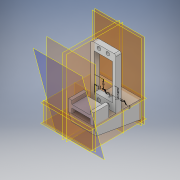
# Autodesk Inventor part: Motor
Saved by Autodesk Inventor 2019.4 (Build 234330000, 330)
## iProperties
Created: 2019-08-20
Part Number: Motor
Material: Genérico
Document SubType Name: Modeling
Designer: Irene
Density: 1 g/cm^3
Appearance: Valor por defecto
Author: Irene
Autodesk Inventor part; units mm, degrees
ref_plane "Plano de trabajo1" through (0, 0, 23) normal (0, 0, 1) x (1, 0, 0)
sketch "Boceto2" plane through (0, 0, 23) normal (0, 0, 1) x (1, 0, 0)
  line L0 (-3, 10) -> (25, 10)
  line L1 (25, 10) -> (25, 65)
  line L2 (23, 67) -> (-1, 67)
  line L3 (-3, 65) -> (-3, 10)
  line L4 (-3, 10) -> (25, 67) construction
  line L5 (25, 10) -> (-3, 67) construction
  line L6 (21.25, 18.406) -> (0.75, 18.406)
  line L7 (0.75, 18.406) -> (0.75, 58.594)
  line L8 (0.75, 58.594) -> (21.25, 58.594)
  line L9 (21.25, 58.594) -> (21.25, 18.406)
  line L10 (21.25, 18.406) -> (0.75, 58.594) construction
  line L11 (0.75, 18.406) -> (21.25, 58.594) construction
  circle A0 centre (6, 63.5) radius 2
  circle A1 centre (16, 63.5) radius 2
  circle A2 centre (6, 13.5) radius 2
  circle A3 centre (16, 13.5) radius 2
  line L12 (25, -6.6) -> (-3, -6.6)
  line L13 (-3, -6.6) -> (-3, 10)
  line L14 (-3, 10) -> (25, 10)
  line L15 (25, 10) -> (25, -6.6)
  line L16 (25, -6.6) -> (-3, 10) construction
  line L17 (-3, -6.6) -> (25, 10) construction
  arc A4 (-1, 67) -> (-3, 65) centre (-1, 65) ccw
  arc A5 (25, 65) -> (23, 67) centre (23, 65) ccw
  point P0 (0, 0)
  point P1 (11, 38.5)
  point P2 (11, 1.7)
  dimension "d5" = 28
  dimension "d6" = 57
  dimension "d9" = 67
  dimension "d10" = 10
  dimension "d12" = 25
  dimension "d13" = 20.5
  dimension "d14" = 40.188
  dimension "d15" = 4
  dimension "d16" = 4
  dimension "d17" = 4
  dimension "d18" = 4
  dimension "d21" = 10
  dimension "d22" = 10
  dimension "d23" = 7
  dimension "d26" = 3.5
  dimension "d27" = 3.5
  dimension "d28" = 3.5
  dimension "d29" = 3.5
  dimension "d38" = 28
  dimension "d39" = 16.6
  dimension "d40" = 25
  dimension "d41" = 10
  dimension "d82" = 2
  dimension "d84" = 7
  dimension "d85" = 9
  constraints: 36 end point, 6 centre point, 6 midpoint, 6 parallel, 4 point on circle, 4 point on line, 4 tangent, 3 horizontal, 3 perpendicular, 1 equal radius
  measures "d5" distance of L5.end L4.end
  measures "d6" distance of L4.end L0.end
  measures "d9" distance from line of point (0, 0) L2
  measures "d10" distance from line of L0 point (0, 0)
  measures "d12" distance from line of L1 point (0, 0)
  measures "d13" distance of L7.end L8.end
  measures "d14" distance of L8.end L6.start
  measures "d15" diameter of A0
  measures "d16" diameter of A1
  measures "d17" diameter of A2
  measures "d18" diameter of A3
  measures "d21" distance of A1.centre A0.centre
  measures "d22" distance of A2.centre A3.centre
  measures "d23" distance edge to line of A2 L3
  measures "d26" distance from line of A2.centre L0
  measures "d27" distance from line of A3.centre L0
  measures "d28" distance from line of A1.centre L2
  measures "d29" distance from line of L2 A0.centre
  measures "d38" distance of L13.end L14.end
  measures "d39" distance of L12.end L13.end
  measures "d40" distance from line of L15 point (0, 0)
  measures "d41" distance from line of L14 point (0, 0)
  measures "d82" radius of A4
  measures "d84" distance edge to line of A1 L1
  measures "d85" distance from line of A0.centre L3
ref_plane "Plano de trabajo2" through (0, 0, 58) normal (0, 0, 1) x (1, 0, 0)
sketch "Boceto3" plane through (0, 0, 58) normal (0, 0, 1) x (1, 0, 0)
  line L0 (25, 0) -> (-3, 0)
  line L1 (-3, 0) -> (-3, 10)
  line L2 (-3, 10) -> (25, 10)
  line L3 (25, 10) -> (25, 0)
  line L4 (25, 0) -> (-3, 10) construction
  line L5 (-3, 0) -> (25, 10) construction
  point P0 (0, 0)
  point P1 (11, 5)
  dimension "d31" = 28
  dimension "d32" = 10
  dimension "d35" = 10
  dimension "d36" = 25
  constraints: 12 end point, 2 midpoint, 2 parallel, 1 horizontal, 1 perpendicular
  measures "d31" distance of L1.end L2.end
  measures "d32" distance of L0.end L1.end
  measures "d35" distance from line of L2 point (0, 0)
  measures "d36" distance from line of L3 point (0, 0)
ref_plane "Plano de trabajo3" through (25, 10, 0) normal (0, 0, 1) x (-1, 0, 0)
sketch "Boceto4" plane through (25, 10, 0) normal (0, 0, 1) x (-1, 0, 0)
  line L0 (0, 0) -> (50, 0)
  line L1 (50, 0) -> (50, 20)
  line L2 (50, 20) -> (0, 20)
  line L3 (0, 20) -> (0, 0)
  line L4 (0, 0) -> (50, 20) construction
  line L5 (50, 0) -> (0, 20) construction
  line L6 (0, 20) -> (0, 0)
  line L7 (28, 0) -> (28, 20)
  point P0 (0, 0)
  dimension "d42" = 50
  dimension "d43" = 20
  dimension "d44" = 50
  dimension "d46" = 28
  constraints: 16 end point, 2 horizontal, 2 parallel, 2 perpendicular, 2 point on line, 2 vertical, 2 other
  measures "d42" distance of L2.end L1.end
  measures "d43" distance of L2.end L0.start
  measures "d44" distance between parallel lines of L1 L6
  measures "d46" distance between parallel lines of L7 L3
ref_plane "Plano de trabajo4" through (25, 10, 0) normal (0, 0, 1) x (-1, 0, 0)
sketch "Boceto5" plane through (25, 10, 0) normal (0, 0, 1) x (-1, 0, 0)
  line L0 (28, 0) -> (28, 20)
  line L1 (28, 20) -> (0, 20)
  line L2 (0, 20) -> (0, 0)
  line L3 (0, 0) -> (28, 0)
  point P0 (25, 10)
  dimension "d48" = 20
  dimension "d49" = 28
  dimension "d50" = 20
  dimension "d51" = 28
  dimension "d52" = 25
  dimension "d53" = 10
  constraints: 8 end point, 2 perpendicular, 1 vertical
  measures "d48" distance of L0.start L0.end
  measures "d49" distance of L0.end L1.end
  measures "d50" distance of L1.end L2.end
  measures "d51" distance of L2.end L0.start
  measures "d52" distance from line of L2 point (25, 10)
  measures "d53" distance from line of L3 point (25, 10)
extrude "Extrusión1" add sketch "Boceto4" along normal blind 3
extrude "Extrusión2" add sketch "Boceto2" along normal blind 6 contours L3 A4 L2 A5 L1 L0
ref_plane "Plano de trabajo5" through (0, 10, 0) normal (0, 1, 0) x (-1, 0, 0)
ref_plane "Plano de trabajo7" through (0, -10, 0) normal (0, 1, 0) x (-1, 0, 0)
loft "Solevación2" add profiles "Boceto3", "Boceto5"
sketch "Boceto9" plane through (0, 10, 0) normal (0, 1, 0) x (-1, 0, 0)
  line L0 (-21.25, 58) -> (-0.75, 58)
  line L1 (-0.75, 58) -> (-0.75, 29)
  line L2 (-0.75, 29) -> (-21.25, 29)
  line L3 (-21.25, 29) -> (-21.25, 58)
  line L4 (-21.25, 58) -> (-0.75, 29) construction
  line L5 (-0.75, 58) -> (-21.25, 29) construction
  line L6 (-23, 29) -> (1, 29) projected
  line L7 (-25, 58) -> (-25, 29) projected
  point P0 (0, 0)
  point P1 (-11, 43.5)
  dimension "d91" = 20.5
  dimension "d92" = 29
  dimension "d93" = 29
  dimension "d94" = 3.75
  constraints: 12 end point, 2 midpoint, 2 parallel, 1 horizontal, 1 perpendicular
  measures "d91" distance of L1.end L2.end
  measures "d92" distance of L0.end L1.end
  measures "d93" distance between parallel lines of L0 L6
  measures "d94" distance between parallel lines of L7 L3
extrude "Extrusión5" add sketch "Boceto9" along normal blind 9
sketch "Boceto10" plane through (0, -10, 0) normal (0, 1, 0) x (-1, 0, 0)
  line L0 (-1, 46) -> (-21, 46)
  line L1 (-21, 46) -> (-21, 3)
  line L2 (-21, 3) -> (-1, 3)
  line L3 (-1, 3) -> (-1, 46)
  line L4 (-1, 46) -> (-21, 3) construction
  line L5 (-21, 46) -> (-1, 3) construction
  line L6 (-25, 58) -> (3, 58) projected
  line L7 (-25, 58) -> (-25, 3) projected
  line L8 (3, 58) -> (3, 3) projected
  line L9 (25, 3) -> (-25, 3) projected
  point P0 (0, 0)
  point P1 (-11, 24.5)
  dimension "d97" = 20
  dimension "d98" = 43
  dimension "d99" = 12
  dimension "d100" = 4
  dimension "d101" = 4
  dimension "d102" = 0
  constraints: 12 end point, 2 midpoint, 2 parallel, 1 horizontal, 1 perpendicular
  measures "d97" distance of L2.end L1.end
  measures "d98" distance of L1.end L0.end
  measures "d99" distance between parallel lines of L0 L6
  measures "d100" distance between parallel lines of L7 L1
  measures "d101" distance between parallel lines of L8 L3
  measures "d102" distance between parallel lines of L9 L2
extrude "Extrusión6" cut sketch "Boceto10" along normal blind 14 contours L3 L2 L1 L0
ref_plane "Plano de trabajo8" through (1, 0, 0) normal (1, 0, 0) x (0, 1, 0)
sketch "Boceto11" plane through (1, 0, 0) normal (1, 0, 0) x (0, 1, 0)
  line L0 (10, 29) -> (24, 29)
  line L1 (24, 29) -> (24, 37)
  line L2 (24, 37) -> (10, 37)
  line L3 (10, 37) -> (10, 29)
  line L4 (10, 29) -> (24, 37) construction
  line L5 (24, 29) -> (10, 37) construction
  line L6 (10, 58) -> (10, 29) projected
  line L7 (65, 29) -> (10, 29) projected
  point P0 (0, 0)
  point P1 (17, 33)
  dimension "d106" = 14
  dimension "d107" = 8
  dimension "d108" = 14
  dimension "d109" = 0
  constraints: 12 end point, 2 midpoint, 2 parallel, 1 horizontal, 1 perpendicular
  measures "d106" distance of L2.end L1.end
  measures "d107" distance of L1.end L0.end
  measures "d108" distance between parallel lines of L6 L1
  measures "d109" distance between parallel lines of L7 L0
extrude "Extrusión7" cut sketch "Boceto11" along normal blind 24 and the other way blind 4
sketch "Boceto12" plane through (-3, 10, 58) normal (0, 1, 0) x (1, 0, 0)
  line L0 (0, 0) -> (0, 21)
  line L1 (3.75, 21) -> (3.75, 0)
  line L2 (3.75, 0) -> (0, 0)
  line L3 (0, 0) -> (0, 21)
  line L4 (35.9308, 19.3547) -> (28, 21)
  line L5 (34.2703, -7.1098) -> (39.6026, 18.5929)
  line L6 (35.9308, 19.3547) -> (39.6026, 18.5929)
  line L7 (39.6026, 18.5929) -> (34.2703, -7.1098)
  line L8 (34.2703, -7.1098) -> (30.5984, -6.348)
  line L9 (3.75, 21) -> (0, 21)
  line L10 (3.75, 21) -> (3.75, 0)
  line L11 (35.9308, 19.3547) -> (30.5984, -6.348)
  line L12 (34.2703, -7.1098) -> (30.5984, -6.348)
  line L13 (3.75, 0) -> (0, 0)
  line L14 (3.75, 21) -> (24.25, 21) projected
  point P0 (18.3993, 70.2266)
  point P1 (0, 21)
  dimension "d130" = 3.75
  dimension "d131" = 0
  constraints: 26 end point, 1 vertical, 3 other
  measures "d130" distance between parallel lines of L1 L0
  measures "d131" distance between parallel lines of L14 L9
extrude "Extrusión9" add sketch "Boceto12" along normal blind 13 contours L0 L9 L1 L2
sketch "Boceto13" plane through (21.25, 10, 58) normal (0, 1, 0) x (1, 0, 0)
  line L0 (3.75, 0) -> (-24.25, 0) projected
  line L1 (3.75, 0) -> (0, 0)
  line L2 (3.75, 0) -> (-1, 0)
  line L3 (-20.5, 0) -> (0, 0) projected
  line L4 (-0.25, 12) -> (-0.25, 55) projected
  line L5 (3.75, 0) -> (3.75, 55) projected
  line L6 (3.75, 0) -> (-1, 0)
  line L7 (0, 0) -> (3.75, 0)
  line L8 (3.75, 0) -> (3.75, 21)
  line L9 (3.75, 21) -> (0, 21)
  line L10 (0, 21) -> (0, 0)
  line L11 (0, 0) -> (3.75, 21) construction
  line L12 (3.75, 0) -> (0, 21) construction
  point P0 (-21.25, 58)
  point P1 (3.75, 21)
  point P2 (0, 21)
  point P3 (1.875, 10.5)
  dimension "d125" = 3.75
  dimension "d126" = 21
  dimension "d127" = 0
  dimension "d128" = 0
  constraints: 18 end point, 2 horizontal, 2 midpoint, 2 parallel, 1 perpendicular, 1 point on line
  measures "d125" distance of L9.end L8.end
  measures "d126" distance of L9.end L7.start
  measures "d127" distance between parallel lines of L0 L7
  measures "d128" distance between parallel lines of L8 L5
extrude "Extrusión10" add sketch "Boceto13" along normal blind 13
ref_plane "Plano de trabajo9" through (-3, 0, 0) normal (1, 0, 0) x (0, 1, 0)
sketch "Boceto14" plane through (-3, 0, 0) normal (1, 0, 0) x (0, 1, 0)
  line L0 (-4, 54) -> (23, 54)
  line L1 (23, 54) -> (23, 58)
  line L2 (23, 58) -> (-4, 58)
  line L3 (-4, 58) -> (-4, 54)
  line L4 (0, 58) -> (23, 58) projected
  line L5 (23, 37) -> (23, 58) projected
  line L6 (10, 37) -> (23, 37) projected
  point P0 (0, 0)
  dimension "d133" = 0
  dimension "d134" = 4
  dimension "d135" = 0
  dimension "d136" = 27
  dimension "d139" = 17
  constraints: 8 end point, 2 parallel, 1 horizontal, 1 perpendicular
  measures "d133" distance between parallel lines of L4 L2
  measures "d134" distance of L0.end L1.end
  measures "d135" distance between parallel lines of L5 L1
  measures "d136" distance of L0.start L0.end
  measures "d139" distance between parallel lines of L0 L6
extrude "Extrusión11" cut sketch "Boceto14" along normal blind 28
ref_plane "Plano de trabajo10" through (0, 0, 54) normal (0, 0, 1) x (1, 0, 0)
sketch "Boceto15" plane through (0, 0, 54) normal (0, 0, 1) x (1, 0, 0)
  line L0 (0.75, 10.0003) -> (21.25, 10.0003)
  line L1 (21.25, 10.0003) -> (21.25, 15.5)
  line L2 (21.25, 15.5) -> (0.75, 15.5)
  line L3 (0.75, 15.5) -> (0.75, 10.0003)
  line L4 (0.75, 18.406) -> (0.75, 58.594) projected
  line L5 (21.25, 58.594) -> (21.25, 18.406) projected
  line L6 (0.75, 19) -> (21.25, 19) projected
  line L7 (25, -0.6897) -> (-3, -0.6897) projected
  point P0 (0, 0)
  dimension "d141" = 0
  dimension "d142" = 0
  dimension "d143" = 3.5
  dimension "d144" = 10.69
  constraints: 8 end point, 2 parallel, 1 horizontal, 1 perpendicular
  measures "d141" distance between parallel lines of L3 L4
  measures "d142" distance between parallel lines of L5 L1
  measures "d143" distance between parallel lines of L6 L2
  measures "d144" distance between parallel lines of L7 L0
extrude "Extrusión12" cut sketch "Boceto15" against normal blind 20
ref_plane "Plano de trabajo11" through (25, 10, 3) normal (0, 0, 1) x (-1, 0, 0)
sketch "Boceto17" plane through (25, 10, 3) normal (0, 0, 1) x (-1, 0, 0)
  circle A0 centre (37.5, 10.5) radius 1.5
  circle A1 centre (15.5, 10.5) radius 1.5
  line L0 (28, 0) -> (50, 0) projected
  line L1 (50, 0) -> (50, 20) projected
  point P0 (25, 10)
  dimension "d154" = 3
  dimension "d155" = 3
  dimension "d156" = 9
  dimension "d157" = 9
  dimension "d158" = 11
  dimension "d159" = 19
  constraints: 2 centre point
  measures "d154" diameter of A0
  measures "d155" diameter of A1
  measures "d156" distance edge to line of A1 L0
  measures "d157" distance edge to line of A0 L0
  measures "d158" distance edge to line of A0 L1
hole "Agujero1" at (-12.5, -0.5, 3) direction (0, 0, -1) diameter 3 end through all
hole "Agujero2" at (9.5, -0.5, 3) direction (0, 0, -1) diameter 3 end through all
ref_plane "Plano de trabajo12" through (9.125, 10.0003, 54) normal (0, 0.2588, -0.9659) x (-1, 0, 0)
sketch "Boceto18" plane through (9.125, 10.0003, 54) normal (0, 0.2588, -0.9659) x (-1, 0, 0)
  line L0 (-15.875, -6.4708) -> (-15.875, 46.6551) projected
  line L1 (16.6517, -12) -> (-15.875, -12)
  line L2 (-15.875, -12) -> (-15.875, 0)
  line L3 (-15.875, 0) -> (16.6517, 0)
  line L4 (16.6517, 0) -> (16.6517, -12)
  line L5 (-12.125, 0) -> (8.375, 0) projected
  point P0 (9.125, -23.6358)
  dimension "d177" = 12
  dimension "d178" = 0
  constraints: 8 end point, 2 parallel, 1 horizontal, 1 perpendicular, 1 point on line
  measures "d177" distance of L1.end L2.end
  measures "d178" distance between parallel lines of L5 L3
extrude "Extrusión13" cut sketch "Boceto18" against normal blind 3.5
